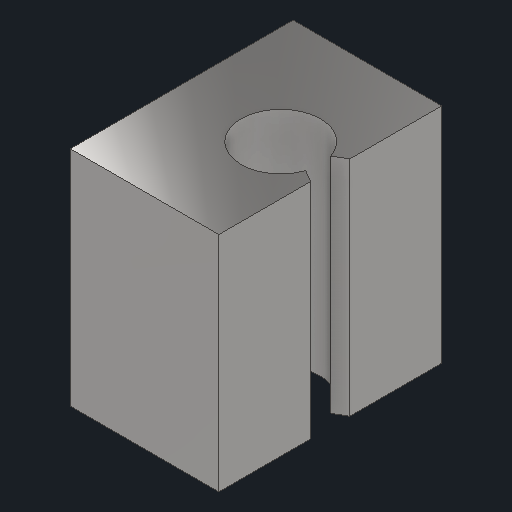
# Autodesk Inventor part: linearbearing
Saved by Autodesk Inventor 2026.3 (Build 303398000, 398)
## iProperties
Created: 2026-06-05
Part Number: linearbearing
Material: ステンレス鋼 440C
Document SubType Name: Modeling
Designer: shusu
Density: 7.75 g/cm^3
Appearance: 半つや出し
Author: shusu
Autodesk Inventor part; units mm, degrees
ref_plane "YZ Plane" through (0, 0, 0) normal (1, 0, 0) x (0, 1, 0)
ref_plane "XZ Plane" through (0, 0, 0) normal (0, 1, 0) x (-1, 0, 0)
ref_plane "XY Plane" through (0, 0, 0) normal (0, 0, 1) x (1, 0, 0)
sketch "スケッチ1" plane through (0, 0, 0) normal (0, 1, 0) x (-1, 0, 0)
  arc A0 (-7.5813, -2.554) -> (-7.5813, 2.554) centre (0, 0) ccw
  line L0 (-10, -3.9505) -> (-7.5813, -2.554)
  line L1 (20, 0) -> (20, -22.5)
  line L2 (20, -22.5) -> (-10, -22.5)
  line L3 (-10, -22.5) -> (-10, -3.9505)
  line L4 (-10, 3.9505) -> (-7.5813, 2.554)
  line L5 (20, 0) -> (20, 22.5)
  line L6 (20, 22.5) -> (-10, 22.5)
  line L7 (-10, 22.5) -> (-10, 3.9505)
  dimension "d4" = 16
  dimension "d8" = 20
  dimension "d9" = 22.5
  dimension "d10" = 30
  constraints: 16 end point, 2 perpendicular, 2 point on circle, 1 centre point, 1 coincident
  measures "d4" diameter of A0
  measures "d8" distance of A0.centre L1.start
  measures "d9" distance of L1.start L1.end
  measures "d10" distance of L1.end L2.end
extrude "押し出し1" add sketch "スケッチ1" along normal blind 45
sketch "スケッチ2" plane through (-20, 0, -22.5) normal (-1, 0, 0) x (0, 0, 1)
  line L0 (45, 0) -> (45, 45) projected
  line L1 (0, 45) -> (45, 45) projected
  line L2 (0, 0) -> (45, 0) projected
  line L3 (22.5, 22.5) -> (22.5, 37.5)
  line L4 (22.5, 37.5) -> (38.5, 37.5)
  line L5 (22.5, 22.5) -> (0, 22.5)
  point P0 (22.5, 0)
  point P1 (6.5, 37.5)
  point P2 (38.5, 7.5)
  point P3 (6.5, 7.5)
  dimension "d13" = 15
  dimension "d14" = 16
  constraints: 6 end point, 3 symmetric about line, 1 coincident, 1 horizontal, 1 perpendicular, 1 vertical
  measures "d13" distance of L3.start L3.end
  measures "d14" distance of L3.end L4.end
hole "穴1" at (-20, 37.5, 16) at (-20, 37.5, -16) at (-20, 7.5, 16) at (-20, 7.5, -16) direction (1, 0, 0) diameter 4.134 depth 10 tip angle 118 thread size "M5x0.8" class "6H" standard "ISO Metric profile"
